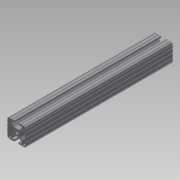
# Autodesk Inventor part: 1504
Saved by Autodesk Inventor 2013 (Build 170138000, 138)
## iProperties
Created: 2014-04-23
Part Number: 1504
Material: Generic
Document SubType Name: Modeling
Density: 1 g/cm^3
Vendor: 80/20 Inc.
Engineer: Ross Bowman
Designer: Ross Bowman
Catalog Web Link: 8020.net
Company: 80/20 Inc.
Author: Ross Bowman
Keywords: 80/20 , 8020 , T-Slot , Extrusion
Material: 6105-T5 Aluminum
Autodesk Inventor part; units mm, degrees
ref_plane "YZ Plane" through (0, 0, 0) normal (1, 0, 0) x (0, 1, 0)
ref_plane "XZ Plane" through (0, 0, 0) normal (0, 1, 0) x (-1, 0, 0)
ref_plane "XY Plane" through (0, 0, 0) normal (0, 0, 1) x (1, 0, 0)
sketch "Sketch1" plane through (0, 0, 0) normal (0, 0, 1) x (1, 0, 0)
  circle A0 centre (0, 0) radius 3.3274
  line L0 (11.1349, 8.9497) -> (8.1479, 5.9632)
  arc A1 (11.1349, 8.9497) -> (12.065, 11.195) centre (8.89, 11.195) ccw
  line L1 (12.065, 16.891) -> (12.065, 11.195)
  arc A2 (12.446, 17.272) -> (12.065, 16.891) centre (12.446, 16.891) ccw
  line L2 (14.478, 17.272) -> (12.446, 17.272)
  arc A3 (17.272, 14.478) -> (14.478, 17.272) centre (14.478, 14.478) ccw
  line L3 (17.272, -14.478) -> (17.272, 14.478)
  arc A4 (14.478, -17.272) -> (17.272, -14.478) centre (14.478, -14.478) ccw
  line L4 (12.446, -17.272) -> (14.478, -17.272)
  arc A5 (12.065, -16.891) -> (12.446, -17.272) centre (12.446, -16.891) ccw
  line L5 (12.065, -11.195) -> (12.065, -16.891)
  arc A6 (12.065, -11.195) -> (11.1349, -8.9497) centre (8.89, -11.195) ccw
  line L6 (8.1479, -5.9632) -> (11.1349, -8.9497)
  arc A7 (6.7564, -2.6043) -> (8.1479, -5.9632) centre (11.5062, -2.6043) ccw
  line L7 (6.7564, 2.6043) -> (6.7564, -2.6043)
  arc A8 (8.1479, 5.9632) -> (6.7564, 2.6043) centre (11.5062, 2.6043) ccw
  line L8 (-12.065, -16.891) -> (-12.065, -11.195)
  arc A9 (-12.446, -17.272) -> (-12.065, -16.891) centre (-12.446, -16.891) ccw
  line L9 (-14.478, -17.272) -> (-12.446, -17.272)
  arc A10 (-17.272, -14.478) -> (-14.478, -17.272) centre (-14.478, -14.478) ccw
  line L10 (-17.272, 14.478) -> (-17.272, -14.478)
  arc A11 (-14.478, 17.272) -> (-17.272, 14.478) centre (-14.478, 14.478) ccw
  line L11 (-12.446, 17.272) -> (-14.478, 17.272)
  arc A12 (-12.065, 16.891) -> (-12.446, 17.272) centre (-12.446, 16.891) ccw
  line L12 (-12.065, 11.195) -> (-12.065, 16.891)
  arc A13 (-12.065, 11.195) -> (-11.1349, 8.9497) centre (-8.89, 11.195) ccw
  line L13 (-8.1479, 5.9632) -> (-11.1349, 8.9497)
  arc A14 (-6.7564, 2.6043) -> (-8.1479, 5.9632) centre (-11.5062, 2.6043) ccw
  line L14 (-6.7564, -2.6043) -> (-6.7564, 2.6043)
  arc A15 (-8.1479, -5.9632) -> (-6.7564, -2.6043) centre (-11.5062, -2.6043) ccw
  line L15 (-11.1349, -8.9497) -> (-8.1479, -5.9632)
  arc A16 (-11.1349, -8.9497) -> (-12.065, -11.195) centre (-8.89, -11.195) ccw
  arc A17 (9.4996, -19.05) -> (7.9756, -19.05) centre (8.7376, -19.05) ccw
  line L16 (9.4996, -19.05) -> (14.3256, -19.05)
  arc A18 (15.8496, -19.05) -> (14.3256, -19.05) centre (15.0876, -19.05) ccw
  line L17 (15.8496, -19.05) -> (15.875, -19.05)
  arc A19 (15.875, -19.05) -> (19.05, -15.875) centre (15.875, -15.875) ccw
  line L18 (19.05, -15.875) -> (19.05, -15.8496)
  arc A20 (19.05, -14.3256) -> (19.05, -15.8496) centre (19.05, -15.0876) ccw
  line L19 (19.05, -14.3256) -> (19.05, -9.4996)
  arc A21 (19.05, -7.9756) -> (19.05, -9.4996) centre (19.05, -8.7376) ccw
  line L20 (19.05, -7.9756) -> (19.05, -0.762)
  arc A22 (19.05, 0.762) -> (19.05, -0.762) centre (19.05, 0) ccw
  line L21 (19.05, 0.762) -> (19.05, 7.9756)
  arc A23 (19.05, 9.4996) -> (19.05, 7.9756) centre (19.05, 8.7376) ccw
  line L22 (19.05, 9.4996) -> (19.05, 14.3256)
  arc A24 (19.05, 15.8496) -> (19.05, 14.3256) centre (19.05, 15.0876) ccw
  line L23 (19.05, 15.8496) -> (19.05, 15.875)
  arc A25 (19.05, 15.875) -> (15.875, 19.05) centre (15.875, 15.875) ccw
  line L24 (15.875, 19.05) -> (15.8496, 19.05)
  arc A26 (14.3256, 19.05) -> (15.8496, 19.05) centre (15.0876, 19.05) ccw
  line L25 (14.3256, 19.05) -> (9.4996, 19.05)
  arc A27 (7.9756, 19.05) -> (9.4996, 19.05) centre (8.7376, 19.05) ccw
  line L26 (7.9756, 19.05) -> (5.6388, 19.05)
  arc A28 (5.6388, 19.05) -> (4.064, 17.4752) centre (5.6388, 17.4752) ccw
  line L27 (4.064, 17.4752) -> (4.064, 16.5608)
  arc A29 (4.064, 16.5608) -> (5.6388, 14.986) centre (5.6388, 16.5608) ccw
  line L28 (5.6388, 14.986) -> (6.4331, 14.986)
  arc A30 (6.4331, 14.986) -> (6.8141, 15.367) centre (6.4331, 15.367) ccw
  line L29 (6.8141, 15.367) -> (6.8141, 15.4437)
  arc A31 (7.1951, 15.8247) -> (6.8141, 15.4437) centre (7.1951, 15.4437) ccw
  line L30 (7.1951, 15.8247) -> (9.017, 15.8247)
  arc A32 (10.287, 14.5547) -> (9.017, 15.8247) centre (9.017, 14.5547) ccw
  line L31 (10.287, 14.5547) -> (10.287, 12.7802)
  arc A33 (10.0267, 12.1519) -> (10.287, 12.7802) centre (9.3985, 12.7802) ccw
  line L32 (10.0267, 12.1519) -> (6.0215, 8.1473)
  arc A34 (2.6631, 6.7564) -> (6.0215, 8.1473) centre (2.6631, 11.5062) ccw
  line L33 (2.6631, 6.7564) -> (-2.6631, 6.7564)
  arc A35 (-6.0215, 8.1473) -> (-2.6631, 6.7564) centre (-2.6631, 11.5062) ccw
  line L34 (-6.0215, 8.1473) -> (-10.0267, 12.1519)
  arc A36 (-10.287, 12.7802) -> (-10.0267, 12.1519) centre (-9.3985, 12.7802) ccw
  line L35 (-10.287, 12.7802) -> (-10.287, 14.5547)
  arc A37 (-9.017, 15.8247) -> (-10.287, 14.5547) centre (-9.017, 14.5547) ccw
  line L36 (-9.017, 15.8247) -> (-7.1951, 15.8247)
  arc A38 (-6.8141, 15.4437) -> (-7.1951, 15.8247) centre (-7.1951, 15.4437) ccw
  line L37 (-6.8141, 15.4437) -> (-6.8141, 15.367)
  arc A39 (-6.8141, 15.367) -> (-6.4331, 14.986) centre (-6.4331, 15.367) ccw
  line L38 (-6.4331, 14.986) -> (-5.6388, 14.986)
  arc A40 (-5.6388, 14.986) -> (-4.064, 16.5608) centre (-5.6388, 16.5608) ccw
  line L39 (-4.064, 16.5608) -> (-4.064, 17.4752)
  arc A41 (-4.064, 17.4752) -> (-5.6388, 19.05) centre (-5.6388, 17.4752) ccw
  line L40 (-5.6388, 19.05) -> (-7.9756, 19.05)
  arc A42 (-9.4996, 19.05) -> (-7.9756, 19.05) centre (-8.7376, 19.05) ccw
  line L41 (-9.4996, 19.05) -> (-14.3256, 19.05)
  arc A43 (-15.8496, 19.05) -> (-14.3256, 19.05) centre (-15.0876, 19.05) ccw
  line L42 (-15.8496, 19.05) -> (-15.875, 19.05)
  arc A44 (-15.875, 19.05) -> (-19.05, 15.875) centre (-15.875, 15.875) ccw
  line L43 (-19.05, 15.875) -> (-19.05, 15.8496)
  arc A45 (-19.05, 14.3256) -> (-19.05, 15.8496) centre (-19.05, 15.0876) ccw
  line L44 (-19.05, 14.3256) -> (-19.05, 9.4996)
  arc A46 (-19.05, 7.9756) -> (-19.05, 9.4996) centre (-19.05, 8.7376) ccw
  line L45 (-19.05, 7.9756) -> (-19.05, 0.762)
  arc A47 (-19.05, -0.762) -> (-19.05, 0.762) centre (-19.05, 0) ccw
  line L46 (-19.05, -0.762) -> (-19.05, -7.9756)
  arc A48 (-19.05, -9.4996) -> (-19.05, -7.9756) centre (-19.05, -8.7376) ccw
  line L47 (-19.05, -9.4996) -> (-19.05, -14.3256)
  arc A49 (-19.05, -15.8496) -> (-19.05, -14.3256) centre (-19.05, -15.0876) ccw
  line L48 (-19.05, -15.8496) -> (-19.05, -15.875)
  arc A50 (-19.05, -15.875) -> (-15.875, -19.05) centre (-15.875, -15.875) ccw
  line L49 (-15.875, -19.05) -> (-15.8496, -19.05)
  arc A51 (-14.3256, -19.05) -> (-15.8496, -19.05) centre (-15.0876, -19.05) ccw
  line L50 (-14.3256, -19.05) -> (-9.4996, -19.05)
  arc A52 (-7.9756, -19.05) -> (-9.4996, -19.05) centre (-8.7376, -19.05) ccw
  line L51 (-7.9756, -19.05) -> (-5.6388, -19.05)
  arc A53 (-5.6388, -19.05) -> (-4.064, -17.4752) centre (-5.6388, -17.4752) ccw
  line L52 (-4.064, -17.4752) -> (-4.064, -16.5608)
  arc A54 (-4.064, -16.5608) -> (-5.6388, -14.986) centre (-5.6388, -16.5608) ccw
  line L53 (-5.6388, -14.986) -> (-6.4331, -14.986)
  arc A55 (-6.4331, -14.986) -> (-6.8141, -15.367) centre (-6.4331, -15.367) ccw
  line L54 (-6.8141, -15.367) -> (-6.8141, -15.4437)
  arc A56 (-7.1951, -15.8247) -> (-6.8141, -15.4437) centre (-7.1951, -15.4437) ccw
  line L55 (-7.1951, -15.8247) -> (-9.017, -15.8247)
  arc A57 (-10.287, -14.5547) -> (-9.017, -15.8247) centre (-9.017, -14.5547) ccw
  line L56 (-10.287, -14.5547) -> (-10.287, -12.7802)
  arc A58 (-10.0267, -12.1519) -> (-10.287, -12.7802) centre (-9.3985, -12.7802) ccw
  line L57 (-10.0267, -12.1519) -> (-6.0215, -8.1473)
  arc A59 (-2.6631, -6.7564) -> (-6.0215, -8.1473) centre (-2.6631, -11.5062) ccw
  line L58 (-2.6631, -6.7564) -> (2.6631, -6.7564)
  arc A60 (6.0215, -8.1473) -> (2.6631, -6.7564) centre (2.6631, -11.5062) ccw
  line L59 (6.0215, -8.1473) -> (10.0267, -12.1519)
  arc A61 (10.287, -12.7802) -> (10.0267, -12.1519) centre (9.3985, -12.7802) ccw
  line L60 (10.287, -12.7802) -> (10.287, -14.5547)
  arc A62 (9.017, -15.8247) -> (10.287, -14.5547) centre (9.017, -14.5547) ccw
  line L61 (9.017, -15.8247) -> (7.1951, -15.8247)
  arc A63 (6.8141, -15.4437) -> (7.1951, -15.8247) centre (7.1951, -15.4437) ccw
  line L62 (6.8141, -15.4437) -> (6.8141, -15.367)
  arc A64 (6.8141, -15.367) -> (6.4331, -14.986) centre (6.4331, -15.367) ccw
  line L63 (6.4331, -14.986) -> (5.6388, -14.986)
  arc A65 (5.6388, -14.986) -> (4.064, -16.5608) centre (5.6388, -16.5608) ccw
  line L64 (4.064, -16.5608) -> (4.064, -17.4752)
  arc A66 (4.064, -17.4752) -> (5.6388, -19.05) centre (5.6388, -17.4752) ccw
  line L65 (5.6388, -19.05) -> (7.9756, -19.05)
  constraints: 132 end point, 132 point on circle, 67 centre point
extrude "Extrusion1" add sketch "Sketch1" against normal blind 304.8
body "Solid1"
